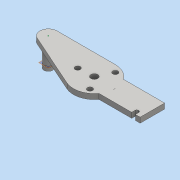
# Autodesk Inventor part: bras-Codeur
Saved by Autodesk Inventor 2016 (Build 200138000, 138)
## iProperties
Created: 2017-02-14
Part Number: bras-Codeur
Material: Generic
Document SubType Name: Modeling
Designer: Aegir
Density: 1 g/cm^3
Appearance: Default
Author: Aegir
Autodesk Inventor part; units mm, degrees
ref_plane "YZ Plane" through (0, 0, 0) normal (1, 0, 0) x (0, 1, 0)
ref_plane "XZ Plane" through (0, 0, 0) normal (0, 1, 0) x (-1, 0, 0)
ref_plane "XY Plane" through (0, 0, 0) normal (0, 0, 1) x (1, 0, 0)
sketch "Esquisse1" plane through (0, 0, 0) normal (0, 0, 1) x (1, 0, 0)
  circle A0 centre (0, 0) radius 2.5 projected
  circle A1 centre (33.5, -7) radius 12 projected
  circle A2 centre (33.5, -7) radius 2 projected
  circle A3 centre (38.485, -14.4933) radius 1.5 projected
  circle A4 centre (24.5181, -7.5705) radius 1.5 projected
  circle A5 centre (37.4969, 1.0638) radius 1.5 projected
  line L0 (0, 5) -> (33.5, 5)
  line L1 (29.0343, -18.1381) -> (-2.5, -4.0756)
  arc A6 (29.0343, -18.1381) -> (33.5, 5) centre (33.5, -7) ccw
  arc A7 (0, 5) -> (-2.5, -4.0756) centre (0, 0.1179) ccw
  circle A8 centre (0, 0.1179) radius 2.4972
  circle A9 centre (37.4969, 1.0638) radius 1.5
  circle A10 centre (24.5181, -7.5705) radius 1.5
  circle A11 centre (38.485, -14.4933) radius 1.5
  constraints: 6 centre point, 6 point on circle, 4 coincident, 4 concentric, 4 end point, 2 tangent, 1 horizontal
extrude "Extrusion1" add sketch "Esquisse1" along normal blind 3 contours A1 L1 | A1 L1 A7 L0 picked at (27.6177, -3.3612)
sketch "Esquisse2" plane through (0, 0, 3) normal (0, 0, 1) x (1, 0, 0)
  point P0 (0, 0)
sketch "Esquisse3" plane through (0, 0, 3) normal (0, 0, 1) x (1, 0, 0)
  line L0 (42.9839, -14.0611) -> (66.9147, -14.0611)
  line L1 (66.9147, -14.0611) -> (66.9147, 0)
  line L2 (66.9147, 0) -> (42.9839, 0)
  circle A0 centre (33.5, -7) radius 2 projected
  circle A1 centre (37.4969, 1.0638) radius 1.5 projected
  circle A2 centre (24.5181, -7.5705) radius 1.5 projected
  circle A3 centre (38.485, -14.4933) radius 1.5 projected
  arc A4 (-2.4972, 0.1179) -> (2.4972, 0.1179) centre (0, 0) ccw projected
  arc A5 (2.4972, 0.1179) -> (-2.4972, 0.1179) centre (0, 0.1179) ccw projected
  arc A6 (0, 5) -> (-2.5, -4.0756) centre (0, 0.1179) ccw projected
  line L3 (-2.5, -4.0756) -> (29.0343, -18.1381) projected
  arc A7 (29.0343, -18.1381) -> (33.5, 5) centre (33.5, -7) ccw projected
  line L4 (33.5, 5) -> (0, 5) projected
  arc A8 (42.9839, -14.0611) -> (42.9839, 0) centre (34.4207, -7.0306) ccw
  constraints: 6 end point, 2 point on circle, 1 centre point, 1 horizontal, 1 parallel, 1 perpendicular
extrude "Extrusion2" add sketch "Esquisse3" against normal blind 3 contours A8 A7 L0 | A7 L2 L1 L0 | A8 L2 A7
sketch "Esquisse4" plane through (0, 0, 0) normal (0, 0, -1) x (-1, 0, 0)
  point P0 (0, 0)
sketch "Esquisse9" plane through (0, 0, 3) normal (0, 0, 1) x (1, 0, 0)
  arc A0 (-2.4972, 0.1179) -> (2.4972, 0.1179) centre (0, 0) ccw projected
  arc A1 (2.4972, 0.1179) -> (-2.4972, 0.1179) centre (0, 0.1179) ccw projected
extrude "Extrusion6" add sketch "Esquisse9" against normal blind 16
ref_plane "Plan de construction1" through (0, 0, -10.3) normal (0, 0, -1) x (-1, 0, 0)
sketch "Esquisse13" plane through (0, 0, -13) normal (0, 0, -1) x (-1, 0, 0)
  circle A0 centre (0, 0) radius 2.932
  constraints: 1 centre point, 1 coincident
extrude "Extrusion8" cut sketch "Esquisse13" against normal up to surface (2.7 mm away)
sketch "Esquisse14" plane through (0, 0, -10.3) normal (0, 0, -1) x (-1, 0, 0)
  circle A0 centre (0, 0) radius 2
  dimension "d20" = 4
  constraints: 1 centre point, 1 coincident
  measures "d20" diameter of A0
extrude "Extrusion9" add sketch "Esquisse14" along normal blind 0.6
sketch "Esquisse15" plane through (0, 0, -10.9) normal (0, 0, -1) x (-1, 0, 0)
  circle A0 centre (0, 0) radius 2.5
  constraints: 1 centre point, 1 coincident
extrude "Extrusion10" add sketch "Esquisse15" along normal blind 2
sketch "Esquisse16" plane through (0, 0, 0) normal (0, 0, -1) x (-1, 0, 0)
  line L0 (-66.9147, -14.0611) -> (-43.2026, -14.0611) projected
  line L1 (-64.1915, -14.0611) -> (-62.052, -14.0611)
  line L2 (-62.052, -14.0611) -> (-62.052, -12.1455)
  line L3 (-63.052, -11.1455) -> (-63.1915, -11.1455)
  line L4 (-64.1915, -12.1455) -> (-64.1915, -14.0611)
  arc A0 (-62.052, -12.1455) -> (-63.052, -11.1455) centre (-63.052, -12.1455) ccw
  arc A1 (-63.1915, -11.1455) -> (-64.1915, -12.1455) centre (-63.1915, -12.1455) ccw
  point P0 (0, 0)
  dimension "d25" = 1
  constraints: 8 end point, 4 point on circle, 4 tangent, 2 centre point, 2 parallel, 1 equal radius, 1 horizontal, 1 perpendicular, 1 point on line
  measures "d25" radius of A0
extrude "Extrusion11" cut sketch "Esquisse16" against normal blind 10
